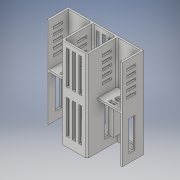
# Autodesk Inventor part: Main_Chassi
Saved by Autodesk Inventor 2018.2 (Build 222227000, 227)
## iProperties
Created: 2018-08-09
Part Number: Main_Chassi
Material: Generic
Document SubType Name: Modeling
Designer: mateu
Density: 1 g/cm^3
Appearance: Default
Author: mateu
Autodesk Inventor part; units mm, degrees
ref_plane "YZ Plane" through (0, 0, 0) normal (1, 0, 0) x (0, 1, 0)
ref_plane "XZ Plane" through (0, 0, 0) normal (0, 1, 0) x (-1, 0, 0)
ref_plane "XY Plane" through (0, 0, 0) normal (0, 0, 1) x (1, 0, 0)
sketch "Sketch1" plane through (0, 0, 0) normal (0, 0, 1) x (1, 0, 0)
  line L0 (0, 0) -> (100, 0)
  line L1 (100, 0) -> (100, 120)
  line L2 (100, 120) -> (0, 120)
  line L3 (0, 120) -> (0, 0)
  dimension "d0" = 100
  dimension "d1" = 120
  constraints: 8 end point, 2 parallel, 1 horizontal, 1 perpendicular
  measures "d0" distance of L2.end L1.end
  measures "d1" distance of L1.end L0.end
extrude "Extrusion1" add sketch "Sketch1" along normal blind 2.4
sketch "Sketch2" plane through (0, 0, 2.4) normal (0, 0, 1) x (1, 0, 0)
  line L0 (0, 120) -> (0, 0) projected
  line L1 (100, 0) -> (100, 120) projected
  line L2 (100, 0) -> (100, 120)
  line L3 (0, 120) -> (0, 0)
  line L4 (97.6, 117.6) -> (97.6, 2.4)
  line L5 (2.4, 2.4) -> (2.4, 117.6)
  line L6 (2.4, 2.4) -> (2.4, 0)
  line L7 (0, 0) -> (100, 0) projected
  line L8 (97.6, 2.4) -> (97.6, 0)
  line L9 (97.6, 117.6) -> (97.6, 120)
  line L10 (2.4, 117.6) -> (2.4, 120)
  line L11 (100, 120) -> (0, 120) projected
  line L12 (97.6, 0) -> (100, 0)
  line L13 (0, 0) -> (2.4, 0)
  line L14 (0, 120) -> (2.4, 120)
  line L15 (97.6, 120) -> (100, 120)
  dimension "d4" = 2.4
  dimension "d5" = 2.4
  constraints: 24 end point, 4 collinear, 3 point on line, 2 parallel, 1 vertical
  measures "d4" distance between parallel lines of L2 L4
  measures "d5" distance between parallel lines of L5 L0
extrude "Extrusion2" add sketch "Sketch2" along normal blind 26 contours L11 L10 L5 L6 L7 L0 | L11 L1 L7 L8 L4 L9
sketch "Sketch3" plane through (0, 0, 2.4) normal (0, 0, 1) x (1, 0, 0)
  line L0 (100, 120) -> (0, 120) projected
  line L1 (0, 0) -> (100, 0) projected
  line L2 (65, 120) -> (67.4, 120)
  line L3 (67.4, 120) -> (67.4, 0)
  line L4 (67.4, 0) -> (65, 0)
  line L5 (65, 0) -> (65, 120)
  line L6 (32.6, 120) -> (35, 120)
  line L7 (35, 120) -> (35, 0)
  line L8 (35, 0) -> (32.6, 0)
  line L9 (32.6, 0) -> (32.6, 120)
  line L10 (50, 120) -> (50, 0)
  dimension "d8" = 2.4
  dimension "d9" = 2.4
  dimension "d10" = 15
  dimension "d11" = 15
  constraints: 18 end point, 4 parallel, 4 point on line, 2 horizontal, 2 midpoint, 2 perpendicular
  measures "d8" distance between parallel lines of L3 L5
  measures "d9" distance between parallel lines of L7 L9
  measures "d10" distance between parallel lines of L10 L7
  measures "d11" distance between parallel lines of L5 L10
extrude "Extrusion3" add sketch "Sketch3" along normal blind 40 contours L3 L1 L5 L0 | L7 L1 L9 L0
sketch "Sketch4" plane through (0, 0, 2.4) normal (0, 0, 1) x (1, 0, 0)
  line L0 (32.6, 0) -> (32.6, 120) projected
  line L1 (2.4, 120) -> (2.4, 0) projected
  line L2 (32.6, 63) -> (2.4, 63)
  line L3 (2.4, 63) -> (2.4, 60.6)
  line L4 (2.4, 60.6) -> (32.6, 60.6)
  line L5 (32.6, 60.6) -> (32.6, 63)
  line L6 (67.4, 0) -> (67.4, 120) projected
  line L7 (97.6, 0) -> (97.6, 120) projected
  line L8 (67.4, 60.6) -> (97.6, 60.6)
  line L9 (97.6, 60.6) -> (97.6, 63)
  line L10 (97.6, 63) -> (67.4, 63)
  line L11 (67.4, 63) -> (67.4, 60.6)
  line L12 (97.6, 120) -> (67.4, 120) projected
  point P0 (0, 0)
  dimension "d14" = 2.4
  dimension "d15" = 57
  constraints: 16 end point, 6 point on line, 4 parallel, 2 horizontal, 2 perpendicular
  measures "d14" distance of L3.end L2.end
  measures "d15" distance between parallel lines of L12 L10
extrude "Extrusion4" add sketch "Sketch4" along normal blind 26 contours L4 L1 L2 L0 | L6 L10 L7 L8
sketch "Sketch5" plane through (2.4, 63, 2.4) normal (0, 1, 0) x (1, 0, 0)
  circle A0 centre (15.1, -13) radius 3.75
  circle A1 centre (80.1, -13) radius 3.75
  line L0 (95.2, 0) -> (65, 0) projected
  line L1 (30.2, 0) -> (0, 0) projected
  line L2 (30.2, 0) -> (30.2, -40) projected
  line L3 (95.2, 0) -> (95.2, -26) projected
  line L4 (11.1, -3) -> (19.1, -3)
  line L5 (19.1, -3) -> (19.1, -7)
  line L6 (19.1, -7) -> (11.1, -7)
  line L7 (11.1, -7) -> (11.1, -3)
  line L8 (76.1, -3) -> (84.1, -3)
  line L9 (84.1, -3) -> (84.1, -7)
  line L10 (84.1, -7) -> (76.1, -7)
  line L11 (76.1, -7) -> (76.1, -3)
  line L12 (76.1, -19) -> (84.1, -19)
  line L13 (84.1, -19) -> (84.1, -23)
  line L14 (84.1, -23) -> (76.1, -23)
  line L15 (76.1, -23) -> (76.1, -19)
  line L16 (11.1, -19) -> (19.1, -19)
  line L17 (19.1, -19) -> (19.1, -23)
  line L18 (19.1, -23) -> (11.1, -23)
  line L19 (11.1, -23) -> (11.1, -19)
  line L20 (0, 0) -> (0, -26) projected
  point P0 (-2.4, 2.4)
  dimension "d18" = 7.5
  dimension "d19" = 7.5
  dimension "d20" = 13
  dimension "d21" = 13
  dimension "d22" = 15.1
  dimension "d23" = 15.1
  dimension "d24" = 4
  dimension "d25" = 4
  dimension "d26" = 8
  dimension "d27" = 8
  dimension "d28" = 8
  dimension "d29" = 4
  dimension "d30" = 8
  dimension "d31" = 4
  dimension "d32" = 6
  dimension "d33" = 11.1
  dimension "d34" = 6
  dimension "d35" = 11.1
  dimension "d36" = 6
  dimension "d37" = 11.1
  dimension "d38" = 11.1
  constraints: 32 end point, 8 parallel, 4 horizontal, 4 perpendicular, 2 centre point, 1 point on line
  measures "d18" diameter of A0
  measures "d19" diameter of A1
  measures "d20" distance from line of L0 A1.centre
  measures "d21" distance from line of L1 A0.centre
  measures "d22" distance from line of L2 A0.centre
  measures "d23" distance from line of L3 A1.centre
  measures "d24" distance of L4.end L5.end
  measures "d25" distance of L8.end L9.end
  measures "d26" distance of L4.start L4.end
  measures "d27" distance of L8.start L8.end
  measures "d28" distance of L13.end L14.end
  measures "d29" distance of L12.end L13.end
  measures "d30" distance of L17.end L18.end
  measures "d31" distance of L16.end L17.end
  measures "d32" distance from line of A0.centre L6
  measures "d33" distance between parallel lines of L20 L7
  measures "d34" distance from line of A0.centre L16
  measures "d35" distance between parallel lines of L2 L17
  measures "d36" distance from line of A1.centre L10
  measures "d37" distance between parallel lines of L3 L9
  measures "d38" distance between parallel lines of L3 L13
extrude "Extrusion5" cut sketch "Sketch5" against normal blind 2.4
sketch "Sketch6" plane through (65, 0, 2.4) normal (-1, 0, 0) x (0, 0, 1)
  line L0 (40, 120) -> (40, 0) projected
  line L1 (0, 0) -> (40, 0) projected
  line L2 (40, 120) -> (37.6, 120)
  line L3 (37.6, 120) -> (37.6, 0)
  line L4 (37.6, 0) -> (40, 0)
  line L5 (40, 0) -> (40, 120)
  point P0 (-2.4, 0)
  dimension "d41" = 2.4
  constraints: 8 end point, 2 parallel, 1 horizontal, 1 perpendicular, 1 point on line
  measures "d41" distance of L4.end L3.end
extrude "Extrusion6" add sketch "Sketch6" along normal blind 32.4
sketch "Sketch8" plane through (0, 0, 2.4) normal (0, 0, 1) x (1, 0, 0)
  line L0 (71.6, 55) -> (93.6, 55)
  line L1 (6.4, 55) -> (28.4, 55)
  line L2 (97.6, 0) -> (97.6, 60.6) projected
  line L3 (2.4, 0) -> (2.4, 60.6) projected
  line L4 (71.6, 7.0064) -> (93.6, 7.0064)
  line L5 (71.6, 7.0064) -> (71.6, 55)
  line L6 (93.6, 55) -> (93.6, 7.0064)
  line L7 (28.4, 7.0064) -> (6.4, 7.0064)
  line L8 (28.4, 7.0064) -> (28.4, 55)
  line L9 (6.4, 55) -> (6.4, 7.0064)
  dimension "d52" = 22
  dimension "d54" = 22
  constraints: 16 end point, 2 parallel, 2 vertical
  measures "d52" distance of L0.start L0.end
  measures "d54" distance of L1.start L1.end
extrude "Extrusion8" cut sketch "Sketch8" against normal blind 2.4
sketch "Sketch9" plane through (0, 0, 0) normal (-1, 0, 0) x (0, 0, 1)
  line L0 (11.65, 63) -> (19.15, 63) projected
  line L1 (19.4, 23) -> (19.4, 51)
  line L2 (19.4, 51) -> (19.4, 11)
  line L3 (19.4, 11) -> (11.4, 11)
  line L4 (11.4, 11) -> (11.4, 51)
  line L5 (11.4, 51) -> (19.4, 51)
  point P0 (0, 0)
  dimension "d64" = 40
  dimension "d65" = 8
  dimension "d132" = 12
  constraints: 10 end point, 2 perpendicular, 1 horizontal, 1 point on line
  measures "d64" distance of L1.end L2.end
  measures "d65" distance of L2.end L3.end
  measures "d132" distance between parallel lines of L0 L5
extrude "Extrusion9" cut sketch "Sketch9" against normal blind 120
fillet "Fillet3" radius 2 1 edges at (2.4, 30.3, 2.4)
fillet "Fillet4" radius 2 1 edges at (97.6, 30.3, 2.4)
fillet "Fillet5" radius 2 1 edges at (35, 60, 2.4)
fillet "Fillet6" radius 2 1 edges at (65, 60, 2.4)
fillet "Fillet7" radius 2 1 edges at (65, 60, 40)
fillet "Fillet8" radius 2 1 edges at (35, 60, 40)
sketch "Sketch14" plane through (0, 0, 0) normal (-1, 0, 0) x (0, 0, 1)
  point P0 (0, 0)
chamfer "Chamfer1" distance 2 angle 45 2 edges at (67.4, 60, 42.4) (32.6, 60, 42.4)
sketch "Sketch15" plane through (0, 0, 0) normal (-1, 0, 0) x (0, 0, 1)
  line L0 (22.406, 110.0269) -> (10.406, 110.0269)
  line L1 (10.406, 110.0269) -> (10.406, 107.0269)
  line L2 (10.406, 107.0269) -> (22.406, 107.0269)
  line L3 (22.406, 107.0269) -> (22.406, 110.0269)
  line L4 (22.406, 102.0269) -> (10.406, 102.0269)
  line L5 (10.406, 102.0269) -> (10.406, 99.0269)
  line L6 (10.406, 99.0269) -> (22.406, 99.0269)
  line L7 (22.406, 99.0269) -> (22.406, 102.0269)
  line L8 (22.406, 94.0269) -> (10.406, 94.0269)
  line L9 (10.406, 94.0269) -> (10.406, 91.0269)
  line L10 (10.406, 91.0269) -> (22.406, 91.0269)
  line L11 (22.406, 91.0269) -> (22.406, 94.0269)
  line L12 (22.406, 86.0269) -> (10.406, 86.0269)
  line L13 (10.406, 86.0269) -> (10.406, 83.0269)
  line L14 (10.406, 83.0269) -> (22.406, 83.0269)
  line L15 (22.406, 83.0269) -> (22.406, 86.0269)
  line L16 (22.406, 78.0269) -> (10.406, 78.0269)
  line L17 (10.406, 78.0269) -> (10.406, 75.0269)
  line L18 (10.406, 75.0269) -> (22.406, 75.0269)
  line L19 (22.406, 75.0269) -> (22.406, 78.0269)
  point P0 (0, 0)
  dimension "d92" = 12
  dimension "d93" = 3
  dimension "d94" = 12
  dimension "d95" = 3
  dimension "d96" = 3
  dimension "d97" = 3
  dimension "d98" = 12
  dimension "d99" = 3
  dimension "d100" = 5
  dimension "d101" = 5
  dimension "d102" = 5
  dimension "d103" = 5
  constraints: 40 end point, 10 parallel, 5 horizontal, 5 perpendicular, 4 point on line
  measures "d92" distance of L2.end L1.end
  measures "d93" distance of L1.end L0.end
  measures "d94" distance of L6.end L5.end
  measures "d95" distance of L5.end L4.end
  measures "d96" distance of L9.end L8.end
  measures "d97" distance of L13.end L12.end
  measures "d98" distance of L18.end L17.end
  measures "d99" distance of L17.end L16.end
  measures "d100" distance between parallel lines of L16 L14
  measures "d101" distance between parallel lines of L10 L12
  measures "d102" distance between parallel lines of L6 L8
  measures "d103" distance between parallel lines of L2 L4
extrude "Extrusion14" cut sketch "Sketch15" against normal blind 120
sketch "Sketch16" plane through (0, 0, 42.4) normal (0, 0, 1) x (1, 0, 0)
  line L0 (52.4, 114.2168) -> (47.6, 114.2168)
  line L1 (47.6, 114.2168) -> (47.6, 69.2168)
  line L2 (47.6, 69.2168) -> (52.4, 69.2168)
  line L3 (52.4, 69.2168) -> (52.4, 114.2168)
  line L4 (60.4, 114.2168) -> (56.4, 114.2168)
  line L5 (56.4, 114.2168) -> (56.4, 69.2168)
  line L6 (56.4, 69.2168) -> (60.4, 69.2168)
  line L7 (60.4, 69.2168) -> (60.4, 114.2168)
  line L8 (43.6, 114.2168) -> (39.6, 114.2168)
  line L9 (39.6, 114.2168) -> (39.6, 69.2168)
  line L10 (39.6, 69.2168) -> (43.6, 69.2168)
  line L11 (43.6, 69.2168) -> (43.6, 114.2168)
  line L12 (60.4, 57.2168) -> (56.4, 57.2168)
  line L13 (56.4, 57.2168) -> (56.4, 12.2168)
  line L14 (56.4, 12.2168) -> (60.4, 12.2168)
  line L15 (60.4, 12.2168) -> (60.4, 57.2168)
  line L16 (52.4, 57.2168) -> (47.6, 57.2168)
  line L17 (47.6, 57.2168) -> (47.6, 12.2168)
  line L18 (47.6, 12.2168) -> (52.4, 12.2168)
  line L19 (52.4, 12.2168) -> (52.4, 57.2168)
  line L20 (43.6, 57.2168) -> (39.6, 57.2168)
  line L21 (39.6, 57.2168) -> (39.6, 12.2168)
  line L22 (39.6, 12.2168) -> (43.6, 12.2168)
  line L23 (43.6, 12.2168) -> (43.6, 57.2168)
  line L24 (65.4, 120) -> (65.4, 0) projected
  line L25 (34.6, 0) -> (34.6, 120) projected
  point P0 (0, 0)
  point P1 (65.4, 2)
  point P2 (34.6, 2)
  dimension "d107" = 45
  dimension "d108" = 4
  dimension "d109" = 45
  dimension "d110" = 4
  dimension "d111" = 45
  dimension "d112" = 45
  dimension "d113" = 4
  dimension "d114" = 4
  dimension "d115" = 4
  dimension "d116" = 5
  dimension "d117" = 5
  dimension "d118" = 5
  dimension "d119" = 5
  dimension "d120" = 4
  dimension "d121" = 4
  dimension "d122" = 12
  dimension "d123" = 12
  dimension "d124" = 12
  dimension "d125" = 4
  constraints: 48 end point, 12 parallel, 6 horizontal, 6 perpendicular, 4 point on line
  measures "d107" distance of L1.end L0.end
  measures "d108" distance of L6.end L5.end
  measures "d109" distance of L5.end L4.end
  measures "d110" distance of L10.end L9.end
  measures "d111" distance of L9.end L8.end
  measures "d112" distance of L13.end L12.end
  measures "d113" distance of L22.end L21.end
  measures "d114" distance between parallel lines of L19 L13
  measures "d115" distance between parallel lines of L23 L17
  measures "d116" distance between parallel lines of L24 L15
  measures "d117" distance between parallel lines of L25 L21
  measures "d118" distance between parallel lines of L24 L7
  measures "d119" distance between parallel lines of L25 L9
  measures "d120" distance between parallel lines of L1 L11
  measures "d121" distance between parallel lines of L5 L3
  measures "d122" distance between parallel lines of L6 L12
  measures "d123" distance between parallel lines of L16 L2
  measures "d124" distance between parallel lines of L10 L20
  measures "d125" distance between parallel lines of L13 L15
extrude "Extrusion15" cut sketch "Sketch16" against normal blind 120
fillet "Fillet11" radius 2 1 edges at (32.6, 91.5, 2.4)
fillet "Fillet12" radius 2 1 edges at (67.4, 91.5, 2.4)
sketch "Sketch17" plane through (0, 0, 2.4) normal (0, 0, 1) x (1, 0, 0)
  line L0 (32.6, 0) -> (32.6, 60.6) projected
  line L1 (28.4, 0) -> (28.4, 55) projected
  line L2 (32.6, 51.1291) -> (28.4, 51.1291)
  line L3 (28.4, 51.1291) -> (28.4, 11.1291)
  line L4 (28.4, 11.1291) -> (32.6, 11.1291)
  line L5 (32.6, 11.1291) -> (32.6, 51.1291)
  line L6 (67.4, 51) -> (67.4, 11) projected
  line L7 (71.6, 0) -> (71.6, 55) projected
  line L8 (67.4, 51) -> (71.6, 51)
  line L9 (71.6, 51) -> (71.6, 11)
  line L10 (71.6, 11) -> (67.4, 11)
  line L11 (67.4, 11) -> (67.4, 51)
  point P0 (0, 0)
  dimension "d133" = 40
  dimension "d134" = 40
  constraints: 16 end point, 4 parallel, 3 point on line, 2 horizontal, 2 perpendicular
  measures "d133" distance of L3.end L2.end
  measures "d134" distance of L8.end L9.end
extrude "Extrusion16" add sketch "Sketch17" along normal blind 9
body "Solid1"
